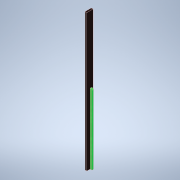
# Autodesk Inventor part: lock4
Saved by Autodesk Inventor 2022 (Build 260153000, 153)
## iProperties
Created: 2021-07-26
Part Number: lock4
Material: Generic
Document SubType Name: Modeling
Designer: Hp
Density: 1 g/cm^3
Appearance: Default
Author: Hp
Autodesk Inventor part; units mm, degrees
ref_plane "YZ Plane" through (0, 0, 0) normal (1, 0, 0) x (0, 1, 0)
ref_plane "XZ Plane" through (0, 0, 0) normal (0, 1, 0) x (-1, 0, 0)
ref_plane "XY Plane" through (0, 0, 0) normal (0, 0, 1) x (1, 0, 0)
sketch "Sketch1" plane through (0, 0, 0) normal (1, 0, 0) x (0, 1, 0)
  line L0 (33.0238, 38.0801) -> (-116.9762, 38.0801)
  line L1 (-116.9762, 38.0801) -> (-116.9762, 31.188)
  line L2 (-116.9762, 31.188) -> (33.0238, 31.188)
  line L3 (33.0238, 31.188) -> (33.0238, 38.0801)
  point P0 (0, 0)
  dimension "d0" = 150
  constraints: 8 end point, 2 parallel, 1 horizontal, 1 perpendicular
  measures "d0" distance of L2.end L1.end
extrude "Extrusion1" add sketch "Sketch1" along normal blind 2
sketch "Sketch2" plane through (2, 0, 0) normal (1, 0, 0) x (0, 0, -1)
  line L0 (-38.0801, -116.9762) -> (-31.188, -116.9762) projected
  line L1 (-34.4927, -40.2559) -> (-32.849, -40.2559)
  line L2 (-32.849, -40.2559) -> (-32.849, -116.9762)
  line L3 (-32.849, -116.9762) -> (-34.4927, -116.9762)
  line L4 (-34.4927, -116.9762) -> (-34.4927, -40.2559)
  point P0 (0, 0)
  constraints: 8 end point, 2 parallel, 1 horizontal, 1 perpendicular, 1 point on line
extrude "Extrusion2" add sketch "Sketch2" along normal blind 2
fillet "Fillet1" radius 1 1 edges at (4, -40.2559, 33.6708)
body "Solid1"
